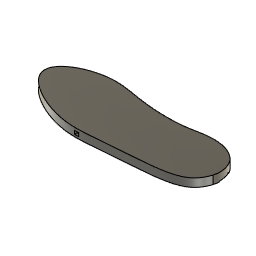
Smart foot brace v1 (Autodesk Fusion 360 design; units mm, degrees)
Autodesk Fusion 360 part; units mm, degrees
note: some values were not read from the file. Set by a fixed rule: which face or edge a step refers to.
sketch "Schizzo2" plane through (0, 0, 0) normal (0, 0, 1) x (1, 0, 0)
  line L0 (-49.9969, 3.1408) -> (-49.9969, -77.002)
  line L1 (269.0032, -13.0421) -> (245.6537, -14.8322)
  line L2 (251.2577, -31.5554) -> (270.315, -30.0944)
  line L3 (270.315, -30.0944) -> (269.0032, -13.0421)
  spline S0 degree 5 poles (239.6431, -39.0842) (239.008, -40.9338) (237.6138, -44.5456) (235.154, -49.7023) (230.6516, -55.9329) (221.1905, -62.1637) (206.5229, -66.4683) (188.36, -69.1663) (168.6133, -70.9116) (148.4991, -72.3278) (128.8774, -73.8918) (110.0255, -75.6871) (91.7256, -77.2705) (73.0453, -77.351) (52.5897, -73.8128) (31.6095, -66.6537) (12.3777, -56.7145) (-2.2618, -45.4213) (-9.8521, -34.1339) (-8.9725, -23.6462) (-0.2666, -13.6017) (14.0848, -4.9823) (31.2393, 1.0769) (48.4813, 3.7209) (63.9221, 3.1001) (77.5489, 1.0443) (90.8033, -1.4303) (105.5547, -3.5848) (122.705, -4.9647) (142.1637, -5.3299) (159.3113, -4.3034) (172.1696, -2.1405) (182.8837, 0.235) (193.8253, 1.7835) (206.3024, 1.6151) (216.9338, -0.4964) (223.8154, -3.6611) (228.407, -6.7709) (231.3167, -9.1532) (232.7333, -10.4216) knots 0 0 0 0 0 0 0.028571 0.057143 0.085714 0.114286 0.142857 0.171429 0.2 0.228571 0.257143 0.285714 0.314286 0.342857 0.371429 0.4 0.428571 0.457143 0.485714 0.514286 0.542857 0.571429 0.6 0.628571 0.657143 0.685714 0.714286 0.742857 0.771429 0.8 0.828571 0.857143 0.885714 0.914286 0.942857 0.971429 1 1 1 1 1 1
  line L4 (247.2731, -16.8633) -> (232.013, -61.305)
  line L5 (235.4873, -58.3623) -> (184.5271, -71.6971)
  line L6 (112.4168, -77.0193) -> (57.595, -77.0134)
  line L7 (-8.4307, -44.1652) -> (-8.4277, -15.72)
  line L8 (26.8163, 3.1326) -> (81.9854, 3.1268)
  line L9 (104.9495, -5.3071) -> (173.0776, -4.7372)
  line L10 (173.2743, 1.9517) -> (226.7543, 0.991)
  line L11 (214.0903, 6.2711) -> (251.3764, -27.1143)
  spline S1 degree 5 poles (239.6431, -39.0842) (239.8525, -38.4743) (240.3443, -37.3331) (241.301, -35.8564) (242.9551, -34.3027) (245.4512, -32.8887) (247.6708, -32.1165) (249.4288, -31.7477) (250.6413, -31.6027) (251.2577, -31.5554) knots 0 0 0 0 0 0 0.2 0.4 0.6 0.8 1 1 1 1 1 1
  spline S2 degree 5 poles (232.7333, -10.4216) (233.164, -10.8072) (234.0487, -11.5321) (235.446, -12.4805) (237.4316, -13.4935) (240.0595, -14.3948) (242.2482, -14.8107) (243.9334, -14.9127) (245.0769, -14.8765) (245.6537, -14.8322) knots 0 0 0 0 0 0 0.2 0.4 0.6 0.8 1 1 1 1 1 1
  line L12 (-8.4292, -101.5202) -> (241.5708, -101.5202)
  line L13 (269.9236, -11.9686) -> (245.5773, -13.8352)
  spline S3 degree 3 poles (233.4004, -9.6766) (235.2721, -11.3525) (237.4456, -12.4757) (239.7715, -13.1715) (241.6374, -13.7297) (243.5687, -13.9891) (245.5773, -13.8352) knots 0 0 0 0 0.554866 0.554866 0.554866 1 1 1 1
  spline S4 degree 3 poles (240.5888, -39.4089) (239.2288, -43.3698) (237.586, -47.1235) (235.258, -50.5942) (233.0296, -53.9163) (230.1256, -56.9559) (226.1195, -59.5307) (222.5382, -61.8324) (218.0521, -63.7558) (212.7264, -65.3147) (204.0376, -67.858) (193.2175, -69.4408) (181.8239, -70.6189) (171.6726, -71.6685) (161.0707, -72.4189) (150.6531, -73.2094) (141.2105, -73.9259) (131.9202, -74.686) (122.8812, -75.4938) (114.5446, -76.2388) (106.4233, -77.0328) (98.2848, -77.5487) (90.3505, -78.0515) (82.3633, -78.2665) (73.9671, -77.5846) (66.6167, -76.9877) (58.9395, -75.6792) (51.1766, -73.6098) (41.5761, -71.0505) (31.86, -67.3391) (23.0777, -62.9007) (14.0271, -58.3266) (6.0213, -53.0215) (0.2781, -47.5919) (-4.7696, -42.8201) (-8.0755, -37.953) (-9.0908, -33.1359) (-9.8586, -29.4927) (-9.2793, -25.8888) (-7.517, -22.488) (-4.7337, -17.1171) (0.9259, -12.1616) (8.0905, -7.9878) (14.6953, -4.1401) (22.5473, -1.0036) (30.4783, 1.0609) (36.8948, 2.7312) (43.3496, 3.689) (49.4389, 4.0032) (55.9944, 4.3414) (62.1106, 3.9625) (67.845, 3.3046) (75.3924, 2.4387) (82.3167, 1.1103) (89.6988, -0.1009) (95.7767, -1.098) (102.2122, -2.0254) (109.3408, -2.7161) (114.6842, -3.2339) (120.4332, -3.6238) (126.4033, -3.8401) (133.1258, -4.0837) (140.0715, -4.0995) (146.4427, -3.8471) (151.9175, -3.6301) (156.9467, -3.2154) (161.4118, -2.663) (169.3887, -1.6762) (175.6132, -0.2481) (181.8504, 0.8561) (185.556, 1.5122) (189.2963, 2.0447) (193.2224, 2.3041) (198.2672, 2.6374) (203.5926, 2.5112) (208.4512, 1.8288) (213.3705, 1.1379) (217.7793, -0.1161) (221.6768, -1.8868) (226.0615, -3.8789) (229.8582, -6.505) (233.4004, -9.6766) knots 0 0 0 0 0.03616105 0.03616105 0.03616105 0.07077455 0.07077455 0.07077455 0.10171712 0.10171712 0.10171712 0.15219932 0.15219932 0.15219932 0.19717723 0.19717723 0.19717723 0.23794526 0.23794526 0.23794526 0.27554534 0.27554534 0.27554534 0.31220121 0.31220121 0.31220121 0.34429112 0.34429112 0.34429112 0.38397767 0.38397767 0.38397767 0.42487674 0.42487674 0.42487674 0.46082195 0.46082195 0.46082195 0.48800841 0.48800841 0.48800841 0.53094375 0.53094375 0.53094375 0.57052484 0.57052484 0.57052484 0.60254726 0.60254726 0.60254726 0.63702043 0.63702043 0.63702043 0.68239288 0.68239288 0.68239288 0.71974977 0.71974977 0.71974977 0.74775154 0.74775154 0.74775154 0.77928259 0.77928259 0.77928259 0.80637744 0.80637744 0.80637744 0.85478308 0.85478308 0.85478308 0.88354135 0.88354135 0.88354135 0.92049365 0.92049365 0.92049365 0.95790815 0.95790815 0.95790815 1 1 1 1
  spline S5 degree 3 poles (240.5888, -39.4089) (241.3059, -37.3208) (242.5674, -35.9265) (244.2133, -34.8517) (245.985, -33.6946) (248.1383, -32.9425) (250.4491, -32.6435) (250.7409, -32.6057) (251.0358, -32.5753) (251.3342, -32.5525) knots 0 0 0 0 0.452012 0.452012 0.452012 0.938578 0.938578 0.938578 1 1 1 1
  line L14 (251.3342, -32.5525) -> (271.3887, -31.015)
  line L15 (271.3887, -31.015) -> (269.9236, -11.9686)
  spline S6 degree 3 poles (243.4498, -40.3145) (243.442, -40.3374) (243.4341, -40.3603) (243.4262, -40.3832) (242.0634, -44.3523) (240.3996, -48.2035) (238.0265, -51.8462) (235.6744, -55.4566) (232.5576, -58.8379) (228.3332, -61.6662) (224.4374, -64.2746) (219.6477, -66.3777) (214.0375, -68.0553) (204.0845, -71.0316) (191.6967, -72.693) (178.8207, -73.9334) (168.6765, -74.9106) (158.2217, -75.637) (148.0073, -76.4198) (138.7072, -77.1325) (129.5865, -77.902) (120.6933, -78.7021) (112.4086, -79.4474) (104.2918, -80.2322) (96.0615, -80.6859) (88.7013, -81.0916) (81.1926, -81.2067) (73.3032, -80.5399) (65.6523, -79.8932) (57.6694, -78.4919) (49.6214, -76.2976) (39.5371, -73.5481) (29.3854, -69.5745) (20.2705, -64.8326) (11.3691, -60.2017) (3.5101, -54.8955) (-2.2653, -49.3107) (-6.7675, -44.9572) (-10.0656, -40.3962) (-11.5628, -35.5397) (-11.7947, -34.7875) (-11.9824, -34.0288) (-12.123, -33.2646) (-12.8162, -29.4949) (-12.2823, -25.6931) (-10.7144, -22.2104) (-8.3374, -16.9306) (-3.8076, -12.3656) (1.8783, -8.3928) (2.4386, -8.0013) (3.0106, -7.6156) (3.5933, -7.2357) (10.8043, -2.5345) (19.6906, 1.2501) (28.7492, 3.7056) (35.3784, 5.5025) (42.0699, 6.5654) (48.4105, 6.9501) (55.1171, 7.3571) (61.376, 7.0246) (67.1852, 6.3967) (74.9752, 5.5546) (82.0081, 4.2133) (89.3533, 2.9966) (95.368, 2.0003) (101.6744, 1.0688) (108.6597, 0.3657) (113.8765, -0.1593) (119.4922, -0.5623) (125.3539, -0.7978) (132.0277, -1.066) (138.9779, -1.1101) (145.3609, -0.8855) (150.7837, -0.6946) (155.782, -0.3097) (160.2056, 0.2129) (167.2628, 1.0468) (172.9356, 2.2385) (178.5539, 3.3007) (182.5227, 4.0511) (186.4973, 4.7256) (190.7246, 5.1154) (195.4849, 5.5543) (200.543, 5.6207) (205.4013, 5.1935) (210.2533, 4.7669) (214.8072, 3.8537) (218.9098, 2.4397) (225.3474, 0.2209) (230.6534, -3.1902) (235.4016, -7.4416) (235.428, -7.4652) (235.4544, -7.4889) (235.4808, -7.5125) knots -0.00020611 -0.00020611 -0.00020611 -0.00020611 0 0 0 0.03482635 0.03482635 0.03482635 0.06918618 0.06918618 0.06918618 0.10083869 0.10083869 0.10083869 0.15703627 0.15703627 0.15703627 0.20132062 0.20132062 0.20132062 0.24164672 0.24164672 0.24164672 0.27922087 0.27922087 0.27922087 0.31279914 0.31279914 0.31279914 0.34534649 0.34534649 0.34534649 0.38613373 0.38613373 0.38613373 0.4259753 0.4259753 0.4259753 0.45704046 0.45704046 0.45704046 0.46185185 0.46185185 0.46185185 0.4854789 0.4854789 0.4854789 0.52150819 0.52150819 0.52150819 0.52505893 0.52505893 0.52505893 0.56895312 0.56895312 0.56895312 0.60106672 0.60106672 0.60106672 0.63505887 0.63505887 0.63505887 0.68067651 0.68067651 0.68067651 0.71802793 0.71802793 0.71802793 0.74591886 0.74591886 0.74591886 0.777679 0.777679 0.777679 0.80466247 0.80466247 0.80466247 0.8477088 0.8477088 0.8477088 0.87807551 0.87807551 0.87807551 0.91224796 0.91224796 0.91224796 0.94637208 0.94637208 0.94637208 1 1 1 1.0003083 1.0003083 1.0003083 1.0003083
  arc A0 (243.4498, -40.3145) -> (235.4808, -7.5125) centre (209.2626, -31.2511) ccw
  point P0 (-8.4292, -29.9426)
  point P1 (54.4009, 3.1297)
  point P2 (139.0136, -5.0221)
  point P3 (200.0143, 1.4714)
  point P4 (85.0059, -77.0164)
  point P5 (210.0072, -65.0297)
  point P6 (85.0059, -77.0164)
  point P7 (85.0059, -81.0152)
  dimension "d6" = 80.1428
  dimension "d10" = 250
  dimension "d15" = 1
  constraint parallel L1 L2
  constraint midpoint S0.start L4
  constraint midpoint P5 L5
  constraint midpoint P6 L6
  constraint midpoint P0 L7
  constraint midpoint P1 L8
  constraint midpoint P2 L9
  constraint midpoint P3 L10
  constraint midpoint S0.end L11
  constraint horizontal L12
  constraint vertical L0
  constraint coincident P6 P4
  constraint coincident S6 P7
  measures "d6" distance of L0.start L0.end
  measures "d10" distance of L12.start L12.end
extrude "Estrusione3" add sketch "Schizzo2" against normal blind 12 contours L11 S2 A0 | L11 S2 S3 S4 A0 | S0 L4 L11 A0 | S0 L10 L11 S4 | L10 L11 S3 S4 S6 A0 | L4 S1 S4 S5 A0 | L4 S1 A0 | S0 L8 L10 S4 | L10 S4 | L10 L11 S4 | S0 L4 L5 S4 | L4 S4 S5 S6 A0 | L7 L10 L11 S4 S6 | L10 L11 S6 | S0 L5 L6 S4 | L5 S4 | L4 L5 S4 S6 | S0 L7 L8 S4 | L8 S4 | S0 L6 L7 S4 | L6 S4 | L5 L7 S4 S6 | L7 S4 | L7 S4 S6
extrude "Estrusione4" [suppressed]
ref_plane "Piano di lavoro1" through (85.0059, -81.0152, 0) normal (-0.000242, -1, 0) x (1, -0.000242, 0)
sketch "Schizzo5" plane through (85.0059, -81.0152, 0) normal (-0.000242, -1, 0) x (1, -0.000242, 0)
  line L0 (158.4341, -12) -> (-97.4394, -12)
  line L1 (-93.4302, 0) -> (156.5698, 0)
  line L2 (6.35, -9.7) -> (-6.35, -9.7)
  line L3 (-6.35, -9.7) -> (-6.35, -3)
  line L4 (-6.35, -3) -> (6.35, -3)
  line L5 (6.35, -3) -> (6.35, -9.7)
  line L6 (3, -8.85) -> (-3, -8.85)
  line L7 (-3, -8.85) -> (-3, -3.85)
  line L8 (-3, -3.85) -> (3, -3.85)
  line L9 (3, -3.85) -> (3, -8.85)
  point P0 (1, -1)
  dimension "d56" = 3
  dimension "d57" = 12.7
  dimension "d58" = 6.7
  dimension "d59" = 6
  dimension "d60" = 5
  dimension "d62" = 0.85
  dimension "d63" = 3.35
  constraint horizontal L2
  constraint vertical L3
  constraint horizontal L4
  constraint vertical L5
  constraint horizontal L6
  constraint vertical L7
  constraint horizontal L8
  constraint vertical L9
  measures "d56" distance of L1 L4
  measures "d57" distance of L3.end L4.end
  measures "d58" distance of L2.start L4.end
  measures "d59" distance of L6.start L6.end
  measures "d60" distance of L6 L8
  measures "d62" distance of L2 L6
  measures "d63" distance of L3 L7
extrude "Estrusione11" cut sketch "Schizzo5" against normal blind 18.5 contours L6 L7 L8 L9
extrude "Estrusione12" cut sketch "Schizzo5" against normal blind 14.5 from surface at -4
extrude "Estrusione13" cut 1 faces at (82.8925, -67.348, -3) along direction (0, 0, -1) blind 20
sketch "Schizzo3" plane through (0, 0, -12) normal (0, 0, -1) x (1, 0, 0)
  arc A0 (235.4808, 7.5125) -> (243.4498, 40.3145) centre (209.2626, 31.2511) ccw
  spline S0 degree 3 poles (243.4498, 40.3145) (243.442, 40.3374) (243.4341, 40.3603) (243.4262, 40.3832) (242.0634, 44.3523) (240.3996, 48.2035) (238.0265, 51.8462) (235.6744, 55.4566) (232.5576, 58.8379) (228.3332, 61.6662) (224.4374, 64.2746) (219.6477, 66.3777) (214.0375, 68.0553) (204.0845, 71.0316) (191.6967, 72.693) (178.8207, 73.9334) (168.6765, 74.9106) (158.2217, 75.637) (148.0073, 76.4198) (138.7072, 77.1325) (129.5865, 77.902) (120.6933, 78.7021) (112.4086, 79.4474) (104.2918, 80.2322) (96.0615, 80.6859) (88.7013, 81.0916) (81.1926, 81.2067) (73.3032, 80.5399) (65.6523, 79.8932) (57.6694, 78.4919) (49.6214, 76.2976) (39.5371, 73.5481) (29.3854, 69.5745) (20.2705, 64.8326) (11.3691, 60.2017) (3.5101, 54.8955) (-2.2653, 49.3107) (-6.7675, 44.9572) (-10.0656, 40.3962) (-11.5628, 35.5397) (-11.7947, 34.7875) (-11.9824, 34.0288) (-12.123, 33.2646) (-12.8162, 29.4949) (-12.2823, 25.6931) (-10.7144, 22.2104) (-8.3374, 16.9306) (-3.8076, 12.3656) (1.8783, 8.3928) (2.4386, 8.0013) (3.0106, 7.6156) (3.5933, 7.2357) (10.8043, 2.5345) (19.6906, -1.2501) (28.7492, -3.7056) (35.3784, -5.5025) (42.0699, -6.5654) (48.4105, -6.9501) (55.1171, -7.3571) (61.376, -7.0246) (67.1852, -6.3967) (74.9752, -5.5546) (82.0081, -4.2133) (89.3533, -2.9966) (95.368, -2.0003) (101.6744, -1.0688) (108.6597, -0.3657) (113.8765, 0.1593) (119.4922, 0.5623) (125.3539, 0.7978) (132.0277, 1.066) (138.9779, 1.1101) (145.3609, 0.8855) (150.7837, 0.6946) (155.782, 0.3097) (160.2056, -0.2129) (167.2628, -1.0468) (172.9356, -2.2385) (178.5539, -3.3007) (182.5227, -4.0511) (186.4973, -4.7256) (190.7246, -5.1154) (195.4849, -5.5543) (200.543, -5.6207) (205.4013, -5.1935) (210.2533, -4.7669) (214.8072, -3.8537) (218.9098, -2.4397) (225.3474, -0.2209) (230.6534, 3.1902) (235.4016, 7.4416) (235.428, 7.4652) (235.4544, 7.4889) (235.4808, 7.5125) knots -0.00020611 -0.00020611 -0.00020611 -0.00020611 0 0 0 0.03482635 0.03482635 0.03482635 0.06918618 0.06918618 0.06918618 0.10083869 0.10083869 0.10083869 0.15703627 0.15703627 0.15703627 0.20132062 0.20132062 0.20132062 0.24164672 0.24164672 0.24164672 0.27922087 0.27922087 0.27922087 0.31279914 0.31279914 0.31279914 0.34534649 0.34534649 0.34534649 0.38613373 0.38613373 0.38613373 0.4259753 0.4259753 0.4259753 0.45704046 0.45704046 0.45704046 0.46185185 0.46185185 0.46185185 0.4854789 0.4854789 0.4854789 0.52150819 0.52150819 0.52150819 0.52505893 0.52505893 0.52505893 0.56895312 0.56895312 0.56895312 0.60106672 0.60106672 0.60106672 0.63505887 0.63505887 0.63505887 0.68067651 0.68067651 0.68067651 0.71802793 0.71802793 0.71802793 0.74591886 0.74591886 0.74591886 0.777679 0.777679 0.777679 0.80466247 0.80466247 0.80466247 0.8477088 0.8477088 0.8477088 0.87807551 0.87807551 0.87807551 0.91224796 0.91224796 0.91224796 0.94637208 0.94637208 0.94637208 1 1 1 1.0003083 1.0003083 1.0003083 1.0003083
  line L0 (-9.581, 38.8184) -> (17.159, 38.8184)
  line L1 (17.159, 38.8184) -> (17.159, 21.0184)
  line L2 (17.159, 21.0184) -> (-9.581, 21.0184)
  line L3 (-9.581, 21.0184) -> (-9.581, 38.8184)
  line L4 (-5.9422, 25.7184) -> (-13.2197, 25.7184)
  line L5 (-13.2197, 25.7184) -> (-13.2197, 34.1184)
  line L6 (-13.2197, 34.1184) -> (-5.9422, 34.1184)
  line L7 (-5.9422, 34.1184) -> (-5.9422, 25.7184)
  line L8 (-5.9422, 25.7184) -> (-13.2197, 34.1184) construction
  line L9 (-13.2197, 25.7184) -> (-5.9422, 34.1184) construction
  line L10 (108.7101, 46.1091) -> (126.2101, 46.1091)
  line L11 (126.2101, 46.1091) -> (126.2101, 15.6091)
  line L12 (126.2101, 15.6091) -> (108.7101, 15.6091)
  line L13 (108.7101, 15.6091) -> (108.7101, 46.1091)
  line L14 (41.4838, 46.1091) -> (93.9838, 46.1091)
  line L15 (93.9838, 46.1091) -> (93.9838, 11.6091)
  line L16 (93.9838, 11.6091) -> (41.4838, 11.6091)
  line L17 (41.4838, 11.6091) -> (41.4838, 46.1091)
  line L18 (140.4408, 46.1091) -> (166.3408, 46.1091)
  line L19 (166.3408, 46.1091) -> (166.3408, 20.7091)
  line L20 (166.3408, 20.7091) -> (140.4408, 20.7091)
  line L21 (140.4408, 20.7091) -> (140.4408, 46.1091)
  line L22 (187.7439, 56.1091) -> (213.6439, 56.1091)
  line L23 (213.6439, 56.1091) -> (213.6439, 7.3491)
  line L24 (213.6439, 7.3491) -> (187.7439, 7.3491)
  line L25 (187.7439, 7.3491) -> (187.7439, 56.1091)
  line L26 (-13.2197, 26.3117) -> (-13.2197, 34.1184)
  line L27 (251.2577, 31.5554) -> (270.315, 30.0944)
  line L28 (270.315, 30.0944) -> (269.0032, 13.0421)
  line L29 (269.0032, 13.0421) -> (245.6537, 14.8322)
  line L30 (270.315, 30.0944) -> (269.0032, 13.0421)
  line L31 (269.0032, 13.0421) -> (209.18, 17.6439)
  line L32 (209.18, 17.6439) -> (210.4917, 34.6962)
  line L33 (210.4917, 34.6962) -> (270.315, 30.0944)
  line L34 (91.3569, 77.0167) -> (91.3604, 62.5167)
  line L35 (91.3604, 62.5167) -> (78.6604, 62.5136)
  line L36 (78.6604, 62.5136) -> (78.6569, 77.0136)
  line L37 (78.6569, 77.0136) -> (91.3569, 77.0167)
  line L38 (187.7439, 56.1091) -> (17.159, 56.1091)
  line L39 (17.159, 56.1091) -> (17.159, 46.1091)
  line L40 (17.159, 46.1091) -> (187.7439, 46.1091)
  line L41 (187.7439, 46.1091) -> (187.7439, 56.1091)
  line L42 (17.159, 46.1091) -> (22.159, 46.1091)
  line L43 (22.159, 46.1091) -> (22.159, 24.9407)
  line L44 (22.159, 24.9407) -> (17.159, 24.9407)
  line L45 (17.159, 24.9407) -> (17.159, 46.1091)
  line L46 (126.2101, 15.6091) -> (108.7101, 15.6091)
  line L47 (108.7101, 15.6091) -> (108.7101, 9.6173)
  line L48 (108.7101, 9.6173) -> (126.2101, 9.6173)
  line L49 (126.2101, 9.6173) -> (126.2101, 15.6091)
  line L50 (91.3604, 62.5167) -> (78.6619, 62.5167)
  line L51 (78.6619, 62.5167) -> (78.6619, 56.1091)
  line L52 (78.6619, 56.1091) -> (91.3604, 56.1091)
  line L53 (91.3604, 56.1091) -> (91.3604, 62.5167)
  point P0 (-9.581, 29.9184)
  dimension "d36" = 26.74
  dimension "d37" = 17.8
  dimension "d38" = 8.4
  dimension "d43" = 30.5
  dimension "d44" = 17.5
  dimension "d45" = 52.5
  dimension "d46" = 34.5
  dimension "d47" = 25.9
  dimension "d48" = 25.4
  dimension "d49" = 25.9
  dimension "d50" = 48.76
  dimension "d88" = 60
  dimension "d92" = 10
  dimension "d93" = 5
  constraint horizontal L0
  constraint vertical L1
  constraint horizontal L2
  constraint vertical L3
  constraint horizontal L4
  constraint perpendicular L4 L5
  constraint parallel L4 L6
  constraint parallel L5 L7
  constraint coincident L8 P0
  constraint coincident L9 P0
  constraint midpoint L3 P0
  constraint horizontal L10
  constraint vertical L11
  constraint horizontal L12
  constraint vertical L13
  constraint horizontal L14
  constraint vertical L15
  constraint horizontal L16
  constraint vertical L17
  constraint horizontal L18
  constraint vertical L19
  constraint horizontal L20
  constraint vertical L21
  constraint horizontal L22
  constraint vertical L23
  constraint horizontal L24
  constraint vertical L25
  constraint vertical L26
  constraint perpendicular L30 L31
  constraint parallel L30 L32
  constraint parallel L31 L33
  constraint coincident L28.end L29.start
  constraint parallel L28 L30
  constraint coincident L27.end L28.start
  constraint horizontal L38
  constraint vertical L39
  constraint horizontal L40
  constraint vertical L41
  constraint collinear L18 L40
  constraint collinear L10 L40
  constraint collinear L14 L40
  constraint collinear L1 L39
  constraint horizontal L42
  constraint vertical L43
  constraint horizontal L44
  constraint vertical L45
  constraint horizontal L46
  constraint vertical L47
  constraint horizontal L48
  constraint vertical L49
  constraint horizontal L50
  constraint vertical L51
  constraint horizontal L52
  constraint vertical L53
  constraint coincident L38 L51.end
  constraint coincident L34.end L35.start
  measures "d36" distance of L0.start L0.end
  measures "d37" distance of L0.start L2.end
  measures "d38" distance of L4.start L6.end
  measures "d43" distance of L10.end L11.end
  measures "d44" distance of L10.start L10.end
  measures "d45" distance of L14.start L14.end
  measures "d46" distance of L14.start L16.end
  measures "d47" distance of L18.start L18.end
  measures "d48" distance of L18.end L19.end
  measures "d49" distance of L22.start L22.end
  measures "d50" distance of L22.start L24.end
  measures "d88" distance of L27.end L32.end
  measures "d92" distance of L38.end L39.end
  measures "d93" distance of L39.end L42.end
extrude "Estrusione USB" cut sketch "Schizzo3" against normal blind 7 contours S0 L4 L5 L6 L26 | S0 L3 L4 L6 | L0 L1 L2 L3 L4 L6 L7 L45 | L3 L4 L6 L7
extrude "Estrusione6" cut sketch "Schizzo3" against normal blind 5 contours L14 L15 L16 L17 L40
extrude "estrusione IMU" cut sketch "Schizzo3" against normal blind 6 contours L18 L19 L20 L21 L40
extrude "Estrusione8" cut sketch "Schizzo3" against normal blind 3 contours L23 L31 L32 L33 | L22 L23 L24 L25 L31 L32 L33 L41
extrude "Estrusione Buck" cut sketch "Schizzo3" against normal blind 8 contours L10 L11 L12 L13 L40 L46
extrude "Estrusione14" cut 3 faces at (213.6439, -28.736, -10) (213.6439, -48.8906, -11) (213.6439, -13.9834, -11) along direction (1, 0, 0) blind 16
extrude "Estrusione15" cut sketch "Schizzo3" against normal blind 1 contours A0 L23 L31 L33
extrude "Estrusione16" cut sketch "Schizzo3" against normal blind 6 contours L10 L14 L18 L25 L38 L39 L40 L41 L42 L52 | L1 L40 L42 L43 L44 L45
extrude "Estrusione17" cut sketch "Schizzo3" against normal blind 8 contours L35 L38 L50 L51 L52 L53
fillet "Raccordo1" radius 2 1 edges at (17.159, -24.9407, -9)
fillet "Raccordo2" radius 2 1 edges at (17.159, -38.8184, -9)
fillet "Raccordo3" radius 2 1 edges at (22.159, -46.1091, -9)
fillet "Raccordo4" radius 2 1 edges at (41.4838, -46.1091, -9.5)
fillet "Raccordo5" radius 2 1 edges at (93.9838, -46.1091, -9.5)
fillet "Raccordo6" radius 2 1 edges at (108.7101, -46.1091, -9)
fillet "Raccordo7" radius 2 1 edges at (126.2101, -46.1091, -9)
fillet "Raccordo8" radius 2 1 edges at (140.4408, -46.1091, -9)
fillet "Raccordo9" radius 2 1 edges at (166.3408, -46.1091, -9)
fillet "Raccordo10" radius 2 1 edges at (187.7439, -46.1091, -10.5)
extrude "Estrusione18" cut sketch "Schizzo3" against normal blind 8 contours L12 L46 L47 L48 L49
equation "MCU_w = 25.4 mm"
equation "MCU_l = 48.26 mm"
equation "MCU_h = 3 mm"
equation "Batt_l = 52 mm"
equation "Batt_w = 34 mm"
equation "Batt_h = 5 mm"
equation "ModRic_l = 28.5 mm"
equation "ModRic_w = 17.3 mm"
equation "ModRic_h = 5 mm"
equation "ModRic_l_onlyboard = 26.24 mm"
equation "IMU_w_l = 25.4 mm"
equation "IMU_h = 6 mm"
equation "Buck_l = 30 mm"
equation "Buck_w = 17 mm"
equation "Buck_h = 8 mm"
equation "d36 = ModRic_l_onlyboard + Hor_tol"
equation "d37 = ModRic_w + Hor_tol"
equation "d38 = USB_c_receptacle"
equation "USB_c_receptacle = 8.4 mm"
equation "d43 = Buck_l + Hor_tol"
equation "d44 = Buck_w + Hor_tol"
equation "d45 = Batt_l + Hor_tol"
equation "d46 = Batt_w + Hor_tol"
equation "d47 = IMU_w_l + Hor_tol"
equation "d48 = IMU_w_l"
equation "d49 = MCU_w + Hor_tol"
equation "d50 = MCU_l + Hor_tol"
equation "Sw_corpo_l = 12.7 mm"
equation "Sw_corpo_w = 6.7 mm"
equation "Sw_pulsante_l = 4 mm"
equation "Sw_pulsante_w = 4 mm"
equation "Sw_pulsante_scorrimento = 6 mm"
equation "d57 = Sw_corpo_l"
equation "d58 = Sw_corpo_w"
equation "d59 = Sw_pulsante_scorrimento"
equation "d62 = ( d58 - d60 ) / 2"
equation "d63 = ( d57 - d59 ) / 2"
equation "d67 = -Batt_h"
equation "d69 = -IMU_h"
equation "d71 = -MCU_h"
equation "d73 = -Buck_h"
equation "Sw_intero_l = 18.5 mm"
equation "d78 = -Sw_intero_l"
equation "d81 = -Sw_pulsante_l"
equation "d82 = -Sw_intero_l + Sw_pulsante_l"
equation "Hor_tol = 0.5 mm"
